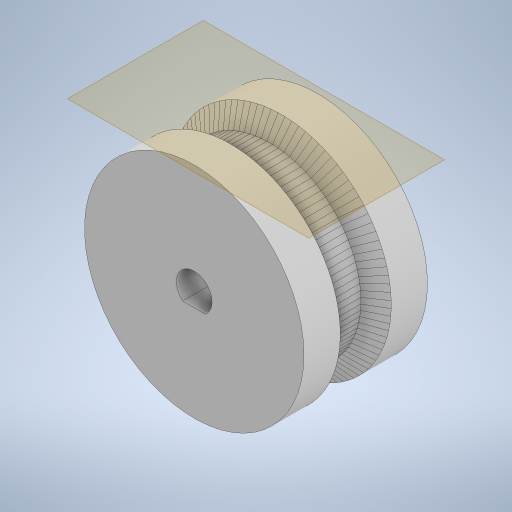
# Autodesk Inventor part: koło
Saved by Autodesk Inventor 2023 (Build 270158000, 158)
## iProperties
Created: 2022-12-13
Part Number: koło
Material: Generic
Document SubType Name: Modeling
Designer: komputer
Density: 1 g/cm^3
Appearance: Default
Author: komputer
Autodesk Inventor part; units mm, degrees
ref_plane "YZ Plane" through (0, 0, 0) normal (1, 0, 0) x (0, 1, 0)
ref_plane "XZ Plane" through (0, 0, 0) normal (0, 1, 0) x (-1, 0, 0)
ref_plane "XY Plane" through (0, 0, 0) normal (0, 0, 1) x (1, 0, 0)
sketch "Sketch1" plane through (0, 0, 0) normal (0, 0, 1) x (1, 0, 0)
  arc A0 (-0.4247, 0.01) -> (-2.6608, 0.01) centre (-1.5427, 1.01) ccw
  arc A1 (-2.6608, 0.01) -> (-0.4247, 0.01) centre (-1.5427, 1.01) ccw
  line L0 (-7.5427, -2.95) -> (-9.5427, -2.95)
  line L1 (-7.5427, 12.35) -> (-7.5427, -2.95)
  line L2 (-7.5427, 12.35) -> (-8.5427, 12.35)
  line L3 (-8.5427, 12.35) -> (-4.5427, 12.35)
  line L4 (-4.5427, 35.8608) -> (-4.5427, 12.35)
  line L5 (1.9573, 15.05) -> (-0.8499, 15.05)
  arc A2 (-2.2355, 15.05) -> (-0.8499, 15.05) centre (-1.5427, 13.95) ccw
  line L6 (-2.2355, 15.05) -> (-5.0427, 15.05)
  arc A3 (-5.0427, 15.05) -> (-5.5427, 14.55) centre (-5.0427, 14.55) ccw
  line L7 (-5.5427, 14.55) -> (-5.5427, 12.85)
  line L8 (-5.5427, 12.85) -> (-7.0427, 12.85)
  arc A4 (-7.0427, 12.85) -> (-7.5427, 12.35) centre (-7.0427, 12.35) ccw
  line L9 (-7.5427, 12.35) -> (-7.5427, -2.45)
  arc A5 (-7.5427, -2.45) -> (-7.0427, -2.95) centre (-7.0427, -2.45) ccw
  line L10 (-7.0427, -2.95) -> (3.9573, -2.95)
  arc A6 (3.9573, -2.95) -> (4.4573, -2.45) centre (3.9573, -2.45) ccw
  line L11 (4.4573, -2.45) -> (4.4573, 12.35)
  arc A7 (4.4573, 12.35) -> (3.9573, 12.85) centre (3.9573, 12.35) ccw
  line L12 (3.9573, 12.85) -> (2.4573, 12.85)
  line L13 (2.4573, 12.85) -> (2.4573, 14.55)
  arc A8 (2.4573, 14.55) -> (1.9573, 15.05) centre (1.9573, 14.55) ccw
  circle A9 centre (-1.5427, 1.01) radius 2
  circle A10 centre (1.2073, 9.85) radius 0.45
  circle A11 centre (0.0302, 6.6603) radius 0.45
  circle A12 centre (-1.5427, 4.59) radius 0.45
  circle A13 centre (2.7073, -1.24) radius 1.25
  circle A14 centre (-5.7927, -1.24) radius 1.25
  line L14 (-1.5427, 1.01) -> (-10.5427, 1.01)
  line L15 (-10.5427, 1.01) -> (-12.5427, 1.01)
  line L16 (-12.5427, 1.01) -> (-9.5427, 1.01)
  circle A15 centre (-1.5427, 1.01) radius 8
  line L17 (-1.5427, 1.01) -> (-1.5427, -6.99)
  line L18 (-1.5427, -6.99) -> (-1.5427, -9.99)
  line L19 (-2.3734, 0.01) -> (-0.7121, 0.01)
  arc A16 (-0.7121, 0.01) -> (-2.3734, 0.01) centre (-1.5427, 1.01) ccw
  line L20 (-8.5427, 12.35) -> (-8.5427, 10.01)
  line L21 (-8.5427, 10.01) -> (-11.5427, 10.01)
  line L22 (-8.5427, 36.4347) -> (-8.5427, 12.35)
  line L23 (-4.5427, 35.8608) -> (-8.5427, 36.4347)
  line L24 (-11.5427, 10.01) -> (-11.5427, -0.95)
  arc A17 (-11.5427, -0.95) -> (-9.5427, -2.95) centre (-9.5427, -0.95) ccw
  point P0 (0, 0)
extrude "Extrusion1" add sketch "Sketch1" against normal blind 9 contours A1 L17 L19 A16 L14 A0 | A0 L14 A9 L17 A1 | L14 A16 L19 L17 A1 A0 | A0 A1 L17 A9 L14 | L14 L1 A15 L11 A6 L10 L17 A9 | A9 L17 L10 A5 L1 L14 | L14 A15 L1 | L1 L0 A15 L14 | L17 A15 L0 L1 A5 L10 | L10 A6 L11 A15 L17 | A11 | A12 | A13 | A14
ref_plane "Płaszczyzna konstrukcyjna1" through (-1.5427, 9.01, 0) normal (0, 1, 0) x (1, 0, 0)
sketch "Szkic2" plane through (-1.5427, 9.01, 0) normal (0, 1, 0) x (1, 0, 0)
  line L0 (8, 9) -> (-8, 9) projected
  line L1 (-8, 0) -> (8, 0) projected
  line L2 (8, 0) -> (8, 9) projected
  line L3 (-8, 0) -> (-8, 9) projected
  line L4 (8, 4.5) -> (6.6434, 4.5)
  line L5 (6.6434, 4.5) -> (6.6434, 5.5)
  line L6 (6.6434, 5.5) -> (6.6434, 3.5)
  line L7 (6.6434, 3.5) -> (8, 2.6389)
  line L8 (6.6434, 5.5) -> (8, 6.3611)
  point P0 (1.5427, 0)
  dimension "d5" = 1
  dimension "d6" = 2
  constraints: 10 end point, 2 point on line, 1 horizontal, 1 midpoint, 1 perpendicular, 1 symmetric about line
  measures "d5" distance of L4.end L5.end
  measures "d6" distance of L5.end L6.end
extrude "Wyciągnięcie proste2" cut sketch "Szkic2" against normal through all contours L2 L4 L5 L8 | L2 L7 L6 L4
pattern_circular "Szyk kołowy1" count 100 over 360 about axis through (-1.5427, 1.01, 0) along (0, 0, -1) of "Wyciągnięcie proste2"
sketch "Szkic3" plane through (-2.3734, 0.01, 0) normal (0, 1, 0) x (1, 0, 0)
  line L0 (1.6613, 0) -> (0, 0) projected
  line L1 (1.6613, 0) -> (1.6613, 9) projected
  line L2 (0, 9) -> (1.6613, 9) projected
  line L3 (0, 0) -> (0, 9) projected
  ellipse E0 centre (0.8307, 1.283) end of major axis (8.8294, 6.356) minor radius 0.2693 (8.8267, 6.3586) -> (8.7952, 6.3586) ccw projected
  line L4 (8.8267, 6.3586) -> (8.8267, 6.3586) projected
  ellipse E1 centre (0.8307, 1.283) end of major axis (8.8294, 6.356) minor radius 0.2693 (8.8267, 6.3586) -> (8.7952, 6.3586) ccw projected
  ellipse E2 centre (0.8307, 1.283) end of major axis (8.8255, 6.3407) minor radius 0.5382 (8.7952, 6.3586) -> (8.7322, 6.3586) ccw projected
  ellipse E3 centre (0.8307, 1.283) end of major axis (8.8191, 6.3151) minor radius 0.8063 (8.7322, 6.3586) -> (8.638, 6.3586) ccw projected
  ellipse E4 centre (0.8307, 1.283) end of major axis (8.8104, 6.279) minor radius 1.0731 (8.638, 6.3586) -> (8.513, 6.3586) ccw projected
  ellipse E5 centre (0.8307, 1.283) end of major axis (8.7994, 6.2323) minor radius 1.3383 (8.513, 6.3586) -> (8.3577, 6.3586) ccw projected
  ellipse E6 centre (0.8307, 1.283) end of major axis (8.7866, 6.1745) minor radius 1.6013 (8.3577, 6.3586) -> (8.1727, 6.3586) ccw projected
  ellipse E7 centre (0.8307, 1.283) end of major axis (8.7721, 6.1054) minor radius 1.8617 (8.1727, 6.3586) -> (7.9587, 6.3586) ccw projected
  ellipse E8 centre (0.8307, 1.283) end of major axis (8.7563, 6.0244) minor radius 2.1191 (7.9587, 6.3586) -> (7.7166, 6.3586) ccw projected
  ellipse E9 centre (0.8307, 1.283) end of major axis (-7.0785, -3.3648) minor radius 2.3729 (7.7166, 6.3586) -> (7.4473, 6.3586) ccw projected
  ellipse E10 centre (0.8307, 1.283) end of major axis (-7.0617, -3.2579) minor radius 2.6225 (7.4473, 6.3586) -> (7.1519, 6.3586) ccw projected
  ellipse E11 centre (0.8307, 1.283) end of major axis (-7.0453, -3.1368) minor radius 2.8673 (7.1519, 6.3586) -> (6.8316, 6.3586) ccw projected
  ellipse E12 centre (0.8307, 1.283) end of major axis (-7.03, -3.0002) minor radius 3.1066 (6.8316, 6.3586) -> (6.4875, 6.3586) ccw projected
  ellipse E13 centre (0.8307, 1.283) end of major axis (-7.0167, -2.8465) minor radius 3.3396 (6.4875, 6.3586) -> (6.1212, 6.3586) ccw projected
  ellipse E14 centre (0.8307, 1.283) end of major axis (-7.0063, -2.6739) minor radius 3.5655 (6.1212, 6.3586) -> (5.7339, 6.3586) ccw projected
  ellipse E15 centre (0.8307, 1.283) end of major axis (-6.9997, -2.48) minor radius 3.7831 (5.7339, 6.3586) -> (5.3273, 6.3586) ccw projected
  ellipse E16 centre (0.8307, 1.283) end of major axis (-6.9981, -2.2621) minor radius 3.9912 (5.3273, 6.3586) -> (4.903, 6.3586) ccw projected
  ellipse E17 centre (0.8307, 1.283) end of major axis (-7.0023, -2.0168) minor radius 4.1884 (4.903, 6.3586) -> (4.4626, 6.3586) ccw projected
  ellipse E18 centre (0.8307, 1.283) end of major axis (-7.0133, -1.7401) minor radius 4.3727 (4.4626, 6.3586) -> (4.0078, 6.3586) ccw projected
  ellipse E19 centre (0.8307, 1.283) end of major axis (-7.0311, -1.4279) minor radius 4.5421 (4.0078, 6.3586) -> (3.5406, 6.3586) ccw projected
  ellipse E20 centre (0.8307, 1.283) end of major axis (-7.0554, -1.0759) minor radius 4.6938 (3.5406, 6.3586) -> (3.0626, 6.3586) ccw projected
  ellipse E21 centre (0.8307, 1.283) end of major axis (-7.0845, -0.6808) minor radius 4.825 (3.0626, 6.3586) -> (2.5758, 6.3586) ccw projected
  ellipse E22 centre (0.8307, 1.283) end of major axis (-7.1152, -0.2416) minor radius 4.9322 (2.5758, 6.3586) -> (2.0821, 6.3586) ccw projected
  ellipse E23 centre (0.8307, 1.283) end of major axis (-7.1428, 0.2388) minor radius 5.012 (2.0821, 6.3586) -> (1.5835, 6.3586) ccw projected
  ellipse E24 centre (0.8307, 1.283) end of major axis (-7.1623, 0.7518) minor radius 5.0614 (1.5835, 6.3586) -> (1.0819, 6.3586) ccw projected
  ellipse E25 centre (0.8307, 1.283) end of major axis (-7.1693, 1.283) minor radius 5.0781 (1.0819, 6.3586) -> (0.5794, 6.3586) ccw projected
  ellipse E26 centre (0.8307, 1.283) end of major axis (8.8236, 0.7518) minor radius 5.0614 (0.5794, 6.3586) -> (0.0778, 6.3586) ccw projected
  ellipse E27 centre (0.8307, 1.283) end of major axis (8.8041, 0.2388) minor radius 5.012 (0.0778, 6.3586) -> (-0.4208, 6.3586) ccw projected
  ellipse E28 centre (0.8307, 1.283) end of major axis (8.7765, -0.2416) minor radius 4.9322 (-0.4208, 6.3586) -> (-0.9145, 6.3586) ccw projected
  ellipse E29 centre (0.8307, 1.283) end of major axis (8.7458, -0.6808) minor radius 4.825 (-0.9145, 6.3586) -> (-1.4013, 6.3586) ccw projected
  ellipse E30 centre (0.8307, 1.283) end of major axis (8.7168, -1.0759) minor radius 4.6938 (-1.4013, 6.3586) -> (-1.8792, 6.3586) ccw projected
  ellipse E31 centre (0.8307, 1.283) end of major axis (8.6924, -1.4279) minor radius 4.5421 (-1.8792, 6.3586) -> (-2.3465, 6.3586) ccw projected
  ellipse E32 centre (0.8307, 1.283) end of major axis (8.6746, -1.7401) minor radius 4.3727 (-2.3465, 6.3586) -> (-2.8013, 6.3586) ccw projected
  ellipse E33 centre (0.8307, 1.283) end of major axis (8.6637, -2.0168) minor radius 4.1884 (-2.8013, 6.3586) -> (-3.2417, 6.3586) ccw projected
  ellipse E34 centre (0.8307, 1.283) end of major axis (8.6594, -2.2621) minor radius 3.9912 (-3.2417, 6.3586) -> (-3.666, 6.3586) ccw projected
  ellipse E35 centre (0.8307, 1.283) end of major axis (8.661, -2.48) minor radius 3.7831 (-3.666, 6.3586) -> (-4.0726, 6.3586) ccw projected
  ellipse E36 centre (0.8307, 1.283) end of major axis (8.6676, -2.6739) minor radius 3.5655 (-4.0726, 6.3586) -> (-4.4598, 6.3586) ccw projected
  ellipse E37 centre (0.8307, 1.283) end of major axis (8.678, -2.8465) minor radius 3.3396 (-4.4598, 6.3586) -> (-4.8262, 6.3586) ccw projected
  ellipse E38 centre (0.8307, 1.283) end of major axis (8.6914, -3.0002) minor radius 3.1066 (-4.8262, 6.3586) -> (-5.1702, 6.3586) ccw projected
  ellipse E39 centre (0.8307, 1.283) end of major axis (8.7066, -3.1368) minor radius 2.8673 (-5.1702, 6.3586) -> (-5.4906, 6.3586) ccw projected
  ellipse E40 centre (0.8307, 1.283) end of major axis (8.723, -3.2579) minor radius 2.6225 (-5.4906, 6.3586) -> (-5.786, 6.3586) ccw projected
  ellipse E41 centre (0.8307, 1.283) end of major axis (8.7398, -3.3648) minor radius 2.3729 (-5.786, 6.3586) -> (-6.0553, 6.3586) ccw projected
  ellipse E42 centre (0.8307, 1.283) end of major axis (8.7563, -3.4583) minor radius 2.1191 (-6.0553, 6.3586) -> (-6.2974, 6.3586) ccw projected
  ellipse E43 centre (0.8307, 1.283) end of major axis (8.7721, -3.5393) minor radius 1.8617 (-6.2974, 6.3586) -> (-6.5114, 6.3586) ccw projected
  ellipse E44 centre (0.8307, 1.283) end of major axis (8.7866, -3.6084) minor radius 1.6013 (-6.5114, 6.3586) -> (-6.6964, 6.3586) ccw projected
  ellipse E45 centre (0.8307, 1.283) end of major axis (8.7994, -3.6662) minor radius 1.3383 (-6.6964, 6.3586) -> (-6.8517, 6.3586) ccw projected
  ellipse E46 centre (0.8307, 1.283) end of major axis (8.8104, -3.713) minor radius 1.0731 (-6.8517, 6.3586) -> (-6.9767, 6.3586) ccw projected
  ellipse E47 centre (0.8307, 1.283) end of major axis (8.8191, -3.7491) minor radius 0.8063 (-6.9767, 6.3586) -> (-7.0708, 6.3586) ccw projected
  ellipse E48 centre (0.8307, 1.283) end of major axis (8.8255, -3.7747) minor radius 0.5382 (-7.0708, 6.3586) -> (-7.1338, 6.3586) ccw projected
  ellipse E49 centre (0.8307, 1.283) end of major axis (8.8294, -3.79) minor radius 0.2693 (-7.1338, 6.3586) -> (-7.1654, 6.3586) ccw projected
  line L5 (-7.1654, 6.3586) -> (-7.1654, 6.3586) projected
  ellipse E50 centre (0.8307, 1.283) end of major axis (8.8294, -3.79) minor radius 0.2693 (-7.1338, 6.3586) -> (-7.1654, 6.3586) ccw projected
  ellipse E51 centre (0.8307, 1.283) end of major axis (8.8255, -3.7747) minor radius 0.5382 (-7.0708, 6.3586) -> (-7.1338, 6.3586) ccw projected
  ellipse E52 centre (0.8307, 1.283) end of major axis (8.8191, -3.7491) minor radius 0.8063 (-6.9767, 6.3586) -> (-7.0708, 6.3586) ccw projected
  ellipse E53 centre (0.8307, 1.283) end of major axis (8.8104, -3.713) minor radius 1.0731 (-6.8517, 6.3586) -> (-6.9767, 6.3586) ccw projected
  ellipse E54 centre (0.8307, 1.283) end of major axis (8.7994, -3.6662) minor radius 1.3383 (-6.6964, 6.3586) -> (-6.8517, 6.3586) ccw projected
  ellipse E55 centre (0.8307, 1.283) end of major axis (8.7866, -3.6084) minor radius 1.6013 (-6.5114, 6.3586) -> (-6.6964, 6.3586) ccw projected
  ellipse E56 centre (0.8307, 1.283) end of major axis (8.7721, -3.5393) minor radius 1.8617 (-6.2974, 6.3586) -> (-6.5114, 6.3586) ccw projected
  ellipse E57 centre (0.8307, 1.283) end of major axis (8.7563, -3.4583) minor radius 2.1191 (-6.0553, 6.3586) -> (-6.2974, 6.3586) ccw projected
  ellipse E58 centre (0.8307, 1.283) end of major axis (-7.0785, 5.9308) minor radius 2.3729 (-5.786, 6.3586) -> (-6.0553, 6.3586) ccw projected
  ellipse E59 centre (0.8307, 1.283) end of major axis (-7.0617, 5.824) minor radius 2.6225 (-5.4906, 6.3586) -> (-5.786, 6.3586) ccw projected
  ellipse E60 centre (0.8307, 1.283) end of major axis (-7.0453, 5.7029) minor radius 2.8673 (-5.1702, 6.3586) -> (-5.4906, 6.3586) ccw projected
  ellipse E61 centre (0.8307, 1.283) end of major axis (-7.03, 5.5662) minor radius 3.1066 (-4.8262, 6.3586) -> (-5.1702, 6.3586) ccw projected
  ellipse E62 centre (0.8307, 1.283) end of major axis (-7.0167, 5.4125) minor radius 3.3396 (-4.4598, 6.3586) -> (-4.8262, 6.3586) ccw projected
  ellipse E63 centre (0.8307, 1.283) end of major axis (-7.0063, 5.2399) minor radius 3.5655 (-4.0726, 6.3586) -> (-4.4598, 6.3586) ccw projected
  ellipse E64 centre (0.8307, 1.283) end of major axis (-6.9997, 5.0461) minor radius 3.7831 (-3.666, 6.3586) -> (-4.0726, 6.3586) ccw projected
  ellipse E65 centre (0.8307, 1.283) end of major axis (-6.9981, 4.8282) minor radius 3.9912 (-3.2417, 6.3586) -> (-3.666, 6.3586) ccw projected
  ellipse E66 centre (0.8307, 1.283) end of major axis (-7.0023, 4.5828) minor radius 4.1884 (-2.8013, 6.3586) -> (-3.2417, 6.3586) ccw projected
  ellipse E67 centre (0.8307, 1.283) end of major axis (-7.0133, 4.3062) minor radius 4.3727 (-2.3465, 6.3586) -> (-2.8013, 6.3586) ccw projected
  ellipse E68 centre (0.8307, 1.283) end of major axis (-7.0311, 3.994) minor radius 4.5421 (-1.8792, 6.3586) -> (-2.3465, 6.3586) ccw projected
  ellipse E69 centre (0.8307, 1.283) end of major axis (-7.0554, 3.642) minor radius 4.6938 (-1.4013, 6.3586) -> (-1.8792, 6.3586) ccw projected
  ellipse E70 centre (0.8307, 1.283) end of major axis (-7.0845, 3.2469) minor radius 4.825 (-0.9145, 6.3586) -> (-1.4013, 6.3586) ccw projected
  ellipse E71 centre (0.8307, 1.283) end of major axis (-7.1152, 2.8076) minor radius 4.9322 (-0.4208, 6.3586) -> (-0.9145, 6.3586) ccw projected
  ellipse E72 centre (0.8307, 1.283) end of major axis (-7.1428, 2.3272) minor radius 5.012 (0.0778, 6.3586) -> (-0.4208, 6.3586) ccw projected
  ellipse E73 centre (0.8307, 1.283) end of major axis (-7.1623, 1.8142) minor radius 5.0614 (0.5794, 6.3586) -> (0.0778, 6.3586) ccw projected
  ellipse E74 centre (0.8307, 1.283) end of major axis (-7.1693, 1.283) minor radius 5.0781 (1.0819, 6.3586) -> (0.5794, 6.3586) ccw projected
  ellipse E75 centre (0.8307, 1.283) end of major axis (8.8236, 1.8142) minor radius 5.0614 (1.5835, 6.3586) -> (1.0819, 6.3586) ccw projected
  ellipse E76 centre (0.8307, 1.283) end of major axis (8.8041, 2.3272) minor radius 5.012 (2.0821, 6.3586) -> (1.5835, 6.3586) ccw projected
  ellipse E77 centre (0.8307, 1.283) end of major axis (8.7765, 2.8076) minor radius 4.9322 (2.5758, 6.3586) -> (2.0821, 6.3586) ccw projected
  ellipse E78 centre (0.8307, 1.283) end of major axis (8.7458, 3.2469) minor radius 4.825 (3.0626, 6.3586) -> (2.5758, 6.3586) ccw projected
  ellipse E79 centre (0.8307, 1.283) end of major axis (8.7168, 3.642) minor radius 4.6938 (3.5406, 6.3586) -> (3.0626, 6.3586) ccw projected
  ellipse E80 centre (0.8307, 1.283) end of major axis (8.6924, 3.994) minor radius 4.5421 (4.0078, 6.3586) -> (3.5406, 6.3586) ccw projected
  ellipse E81 centre (0.8307, 1.283) end of major axis (8.6746, 4.3062) minor radius 4.3727 (4.4626, 6.3586) -> (4.0078, 6.3586) ccw projected
  ellipse E82 centre (0.8307, 1.283) end of major axis (8.6637, 4.5828) minor radius 4.1884 (4.903, 6.3586) -> (4.4626, 6.3586) ccw projected
  ellipse E83 centre (0.8307, 1.283) end of major axis (8.6594, 4.8282) minor radius 3.9912 (5.3273, 6.3586) -> (4.903, 6.3586) ccw projected
  ellipse E84 centre (0.8307, 1.283) end of major axis (8.661, 5.0461) minor radius 3.7831 (5.7339, 6.3586) -> (5.3273, 6.3586) ccw projected
  ellipse E85 centre (0.8307, 1.283) end of major axis (8.6676, 5.2399) minor radius 3.5655 (6.1212, 6.3586) -> (5.7339, 6.3586) ccw projected
  ellipse E86 centre (0.8307, 1.283) end of major axis (8.678, 5.4125) minor radius 3.3396 (6.4875, 6.3586) -> (6.1212, 6.3586) ccw projected
  ellipse E87 centre (0.8307, 1.283) end of major axis (8.6914, 5.5662) minor radius 3.1066 (6.8316, 6.3586) -> (6.4875, 6.3586) ccw projected
  ellipse E88 centre (0.8307, 1.283) end of major axis (8.7066, 5.7029) minor radius 2.8673 (7.1519, 6.3586) -> (6.8316, 6.3586) ccw projected
  ellipse E89 centre (0.8307, 1.283) end of major axis (8.723, 5.824) minor radius 2.6225 (7.4473, 6.3586) -> (7.1519, 6.3586) ccw projected
  ellipse E90 centre (0.8307, 1.283) end of major axis (8.7398, 5.9308) minor radius 2.3729 (7.7166, 6.3586) -> (7.4473, 6.3586) ccw projected
  ellipse E91 centre (0.8307, 1.283) end of major axis (8.7563, 6.0244) minor radius 2.1191 (7.9587, 6.3586) -> (7.7166, 6.3586) ccw projected
  ellipse E92 centre (0.8307, 1.283) end of major axis (8.7721, 6.1054) minor radius 1.8617 (8.1727, 6.3586) -> (7.9587, 6.3586) ccw projected
  ellipse E93 centre (0.8307, 1.283) end of major axis (8.7866, 6.1745) minor radius 1.6013 (8.3577, 6.3586) -> (8.1727, 6.3586) ccw projected
  ellipse E94 centre (0.8307, 1.283) end of major axis (8.7994, 6.2323) minor radius 1.3383 (8.513, 6.3586) -> (8.3577, 6.3586) ccw projected
  ellipse E95 centre (0.8307, 1.283) end of major axis (8.8104, 6.279) minor radius 1.0731 (8.638, 6.3586) -> (8.513, 6.3586) ccw projected
  ellipse E96 centre (0.8307, 1.283) end of major axis (8.8191, 6.3151) minor radius 0.8063 (8.7322, 6.3586) -> (8.638, 6.3586) ccw projected
  ellipse E97 centre (0.8307, 1.283) end of major axis (8.8255, 6.3407) minor radius 0.5382 (8.7952, 6.3586) -> (8.7322, 6.3586) ccw projected
  line L6 (8.8307, 9) -> (-7.1693, 9) projected
  line L7 (-7.1693, 0) -> (8.8307, 0) projected
  ellipse E98 centre (0.8307, 7.717) end of major axis (8.8294, 2.644) minor radius 0.2693 (8.7952, 2.6414) -> (8.8267, 2.6414) ccw projected
  ellipse E99 centre (0.8307, 7.717) end of major axis (8.8255, 2.6593) minor radius 0.5382 (8.7322, 2.6414) -> (8.7952, 2.6414) ccw projected
  ellipse E100 centre (0.8307, 7.717) end of major axis (8.8191, 2.6849) minor radius 0.8063 (8.638, 2.6414) -> (8.7322, 2.6414) ccw projected
  ellipse E101 centre (0.8307, 7.717) end of major axis (8.8104, 2.721) minor radius 1.0731 (8.513, 2.6414) -> (8.638, 2.6414) ccw projected
  ellipse E102 centre (0.8307, 7.717) end of major axis (8.7994, 2.7677) minor radius 1.3383 (8.3577, 2.6414) -> (8.513, 2.6414) ccw projected
  ellipse E103 centre (0.8307, 7.717) end of major axis (8.7866, 2.8255) minor radius 1.6013 (8.1727, 2.6414) -> (8.3577, 2.6414) ccw projected
  ellipse E104 centre (0.8307, 7.717) end of major axis (8.7721, 2.8946) minor radius 1.8617 (7.9587, 2.6414) -> (8.1727, 2.6414) ccw projected
  ellipse E105 centre (0.8307, 7.717) end of major axis (8.7563, 2.9756) minor radius 2.1191 (7.7166, 2.6414) -> (7.9587, 2.6414) ccw projected
  ellipse E106 centre (0.8307, 7.717) end of major axis (-7.0785, 12.3648) minor radius 2.3729 (7.4473, 2.6414) -> (7.7166, 2.6414) ccw projected
  ellipse E107 centre (0.8307, 7.717) end of major axis (-7.0617, 12.2579) minor radius 2.6225 (7.1519, 2.6414) -> (7.4473, 2.6414) ccw projected
  ellipse E108 centre (0.8307, 7.717) end of major axis (-7.0453, 12.1368) minor radius 2.8673 (6.8316, 2.6414) -> (7.1519, 2.6414) ccw projected
  ellipse E109 centre (0.8307, 7.717) end of major axis (-7.03, 12.0002) minor radius 3.1066 (6.4875, 2.6414) -> (6.8316, 2.6414) ccw projected
  ellipse E110 centre (0.8307, 7.717) end of major axis (-7.0167, 11.8465) minor radius 3.3396 (6.1212, 2.6414) -> (6.4875, 2.6414) ccw projected
  ellipse E111 centre (0.8307, 7.717) end of major axis (-7.0063, 11.6739) minor radius 3.5655 (5.7339, 2.6414) -> (6.1212, 2.6414) ccw projected
  ellipse E112 centre (0.8307, 7.717) end of major axis (-6.9997, 11.48) minor radius 3.7831 (5.3273, 2.6414) -> (5.7339, 2.6414) ccw projected
  ellipse E113 centre (0.8307, 7.717) end of major axis (-6.9981, 11.2621) minor radius 3.9912 (4.903, 2.6414) -> (5.3273, 2.6414) ccw projected
  ellipse E114 centre (0.8307, 7.717) end of major axis (-7.0023, 11.0168) minor radius 4.1884 (4.4626, 2.6414) -> (4.903, 2.6414) ccw projected
  ellipse E115 centre (0.8307, 7.717) end of major axis (-7.0133, 10.7401) minor radius 4.3727 (4.0078, 2.6414) -> (4.4626, 2.6414) ccw projected
  ellipse E116 centre (0.8307, 7.717) end of major axis (-7.0311, 10.4279) minor radius 4.5421 (3.5406, 2.6414) -> (4.0078, 2.6414) ccw projected
  ellipse E117 centre (0.8307, 7.717) end of major axis (-7.0554, 10.0759) minor radius 4.6938 (3.0626, 2.6414) -> (3.5406, 2.6414) ccw projected
  ellipse E118 centre (0.8307, 7.717) end of major axis (-7.0845, 9.6808) minor radius 4.825 (2.5758, 2.6414) -> (3.0626, 2.6414) ccw projected
  ellipse E119 centre (0.8307, 7.717) end of major axis (-7.1152, 9.2416) minor radius 4.9322 (2.0821, 2.6414) -> (2.5758, 2.6414) ccw projected
  ellipse E120 centre (0.8307, 7.717) end of major axis (-7.1428, 8.7612) minor radius 5.012 (1.5835, 2.6414) -> (2.0821, 2.6414) ccw projected
  ellipse E121 centre (0.8307, 7.717) end of major axis (-7.1623, 8.2482) minor radius 5.0614 (1.0819, 2.6414) -> (1.5835, 2.6414) ccw projected
  ellipse E122 centre (0.8307, 7.717) end of major axis (8.8307, 7.717) minor radius 5.0781 (0.5794, 2.6414) -> (1.0819, 2.6414) ccw projected
  ellipse E123 centre (0.8307, 7.717) end of major axis (8.8236, 8.2482) minor radius 5.0614 (0.0778, 2.6414) -> (0.5794, 2.6414) ccw projected
  ellipse E124 centre (0.8307, 7.717) end of major axis (8.8041, 8.7612) minor radius 5.012 (-0.4208, 2.6414) -> (0.0778, 2.6414) ccw projected
  ellipse E125 centre (0.8307, 7.717) end of major axis (8.7765, 9.2416) minor radius 4.9322 (-0.9145, 2.6414) -> (-0.4208, 2.6414) ccw projected
  ellipse E126 centre (0.8307, 7.717) end of major axis (8.7458, 9.6808) minor radius 4.825 (-1.4013, 2.6414) -> (-0.9145, 2.6414) ccw projected
  ellipse E127 centre (0.8307, 7.717) end of major axis (8.7168, 10.0759) minor radius 4.6938 (-1.8792, 2.6414) -> (-1.4013, 2.6414) ccw projected
  ellipse E128 centre (0.8307, 7.717) end of major axis (8.6924, 10.4279) minor radius 4.5421 (-2.3465, 2.6414) -> (-1.8792, 2.6414) ccw projected
  ellipse E129 centre (0.8307, 7.717) end of major axis (8.6746, 10.7401) minor radius 4.3727 (-2.8013, 2.6414) -> (-2.3465, 2.6414) ccw projected
  ellipse E130 centre (0.8307, 7.717) end of major axis (8.6637, 11.0168) minor radius 4.1884 (-3.2417, 2.6414) -> (-2.8013, 2.6414) ccw projected
  ellipse E131 centre (0.8307, 7.717) end of major axis (8.6594, 11.2621) minor radius 3.9912 (-3.666, 2.6414) -> (-3.2417, 2.6414) ccw projected
  ellipse E132 centre (0.8307, 7.717) end of major axis (8.661, 11.48) minor radius 3.7831 (-4.0726, 2.6414) -> (-3.666, 2.6414) ccw projected
  ellipse E133 centre (0.8307, 7.717) end of major axis (8.6676, 11.6739) minor radius 3.5655 (-4.4598, 2.6414) -> (-4.0726, 2.6414) ccw projected
  ellipse E134 centre (0.8307, 7.717) end of major axis (8.678, 11.8465) minor radius 3.3396 (-4.8262, 2.6414) -> (-4.4598, 2.6414) ccw projected
  ellipse E135 centre (0.8307, 7.717) end of major axis (8.6914, 12.0002) minor radius 3.1066 (-5.1702, 2.6414) -> (-4.8262, 2.6414) ccw projected
  ellipse E136 centre (0.8307, 7.717) end of major axis (8.7066, 12.1368) minor radius 2.8673 (-5.4906, 2.6414) -> (-5.1702, 2.6414) ccw projected
  ellipse E137 centre (0.8307, 7.717) end of major axis (8.723, 12.2579) minor radius 2.6225 (-5.786, 2.6414) -> (-5.4906, 2.6414) ccw projected
  ellipse E138 centre (0.8307, 7.717) end of major axis (8.7398, 12.3648) minor radius 2.3729 (-6.0553, 2.6414) -> (-5.786, 2.6414) ccw projected
  ellipse E139 centre (0.8307, 7.717) end of major axis (8.7563, 12.4583) minor radius 2.1191 (-6.2974, 2.6414) -> (-6.0553, 2.6414) ccw projected
  ellipse E140 centre (0.8307, 7.717) end of major axis (8.7721, 12.5393) minor radius 1.8617 (-6.5114, 2.6414) -> (-6.2974, 2.6414) ccw projected
  ellipse E141 centre (0.8307, 7.717) end of major axis (8.7866, 12.6084) minor radius 1.6013 (-6.6964, 2.6414) -> (-6.5114, 2.6414) ccw projected
  ellipse E142 centre (0.8307, 7.717) end of major axis (8.7994, 12.6662) minor radius 1.3383 (-6.8517, 2.6414) -> (-6.6964, 2.6414) ccw projected
  ellipse E143 centre (0.8307, 7.717) end of major axis (8.8104, 12.713) minor radius 1.0731 (-6.9767, 2.6414) -> (-6.8517, 2.6414) ccw projected
  ellipse E144 centre (0.8307, 7.717) end of major axis (8.8191, 12.7491) minor radius 0.8063 (-7.0708, 2.6414) -> (-6.9767, 2.6414) ccw projected
  ellipse E145 centre (0.8307, 7.717) end of major axis (8.8255, 12.7747) minor radius 0.5382 (-7.1338, 2.6414) -> (-7.0708, 2.6414) ccw projected
  ellipse E146 centre (0.8307, 7.717) end of major axis (8.8294, 12.79) minor radius 0.2693 (-7.1654, 2.6414) -> (-7.1338, 2.6414) ccw projected
  line L8 (-7.1654, 2.6414) -> (-7.1654, 2.6414) projected
  ellipse E147 centre (0.8307, 7.717) end of major axis (8.8294, 12.79) minor radius 0.2693 (-7.1654, 2.6414) -> (-7.1338, 2.6414) ccw projected
  ellipse E148 centre (0.8307, 7.717) end of major axis (8.8255, 12.7747) minor radius 0.5382 (-7.1338, 2.6414) -> (-7.0708, 2.6414) ccw projected
  ellipse E149 centre (0.8307, 7.717) end of major axis (8.8191, 12.7491) minor radius 0.8063 (-7.0708, 2.6414) -> (-6.9767, 2.6414) ccw projected
  ellipse E150 centre (0.8307, 7.717) end of major axis (8.8104, 12.713) minor radius 1.0731 (-6.9767, 2.6414) -> (-6.8517, 2.6414) ccw projected
  ellipse E151 centre (0.8307, 7.717) end of major axis (8.7994, 12.6662) minor radius 1.3383 (-6.8517, 2.6414) -> (-6.6964, 2.6414) ccw projected
  ellipse E152 centre (0.8307, 7.717) end of major axis (8.7866, 12.6084) minor radius 1.6013 (-6.6964, 2.6414) -> (-6.5114, 2.6414) ccw projected
  ellipse E153 centre (0.8307, 7.717) end of major axis (8.7721, 12.5393) minor radius 1.8617 (-6.5114, 2.6414) -> (-6.2974, 2.6414) ccw projected
  ellipse E154 centre (0.8307, 7.717) end of major axis (8.7563, 12.4583) minor radius 2.1191 (-6.2974, 2.6414) -> (-6.0553, 2.6414) ccw projected
  ellipse E155 centre (0.8307, 7.717) end of major axis (-7.0785, 3.0692) minor radius 2.3729 (-6.0553, 2.6414) -> (-5.786, 2.6414) ccw projected
  ellipse E156 centre (0.8307, 7.717) end of major axis (-7.0617, 3.176) minor radius 2.6225 (-5.786, 2.6414) -> (-5.4906, 2.6414) ccw projected
  ellipse E157 centre (0.8307, 7.717) end of major axis (-7.0453, 3.2971) minor radius 2.8673 (-5.4906, 2.6414) -> (-5.1702, 2.6414) ccw projected
  ellipse E158 centre (0.8307, 7.717) end of major axis (-7.03, 3.4338) minor radius 3.1066 (-5.1702, 2.6414) -> (-4.8262, 2.6414) ccw projected
  ellipse E159 centre (0.8307, 7.717) end of major axis (-7.0167, 3.5875) minor radius 3.3396 (-4.8262, 2.6414) -> (-4.4598, 2.6414) ccw projected
  ellipse E160 centre (0.8307, 7.717) end of major axis (-7.0063, 3.7601) minor radius 3.5655 (-4.4598, 2.6414) -> (-4.0726, 2.6414) ccw projected
  ellipse E161 centre (0.8307, 7.717) end of major axis (-6.9997, 3.9539) minor radius 3.7831 (-4.0726, 2.6414) -> (-3.666, 2.6414) ccw projected
  ellipse E162 centre (0.8307, 7.717) end of major axis (-6.9981, 4.1718) minor radius 3.9912 (-3.666, 2.6414) -> (-3.2417, 2.6414) ccw projected
  ellipse E163 centre (0.8307, 7.717) end of major axis (-7.0023, 4.4172) minor radius 4.1884 (-3.2417, 2.6414) -> (-2.8013, 2.6414) ccw projected
  ellipse E164 centre (0.8307, 7.717) end of major axis (-7.0133, 4.6938) minor radius 4.3727 (-2.8013, 2.6414) -> (-2.3465, 2.6414) ccw projected
  ellipse E165 centre (0.8307, 7.717) end of major axis (-7.0311, 5.006) minor radius 4.5421 (-2.3465, 2.6414) -> (-1.8792, 2.6414) ccw projected
  ellipse E166 centre (0.8307, 7.717) end of major axis (-7.0554, 5.358) minor radius 4.6938 (-1.8792, 2.6414) -> (-1.4013, 2.6414) ccw projected
  ellipse E167 centre (0.8307, 7.717) end of major axis (-7.0845, 5.7531) minor radius 4.825 (-1.4013, 2.6414) -> (-0.9145, 2.6414) ccw projected
  ellipse E168 centre (0.8307, 7.717) end of major axis (-7.1152, 6.1924) minor radius 4.9322 (-0.9145, 2.6414) -> (-0.4208, 2.6414) ccw projected
  ellipse E169 centre (0.8307, 7.717) end of major axis (-7.1428, 6.6728) minor radius 5.012 (-0.4208, 2.6414) -> (0.0778, 2.6414) ccw projected
  ellipse E170 centre (0.8307, 7.717) end of major axis (-7.1623, 7.1858) minor radius 5.0614 (0.0778, 2.6414) -> (0.5794, 2.6414) ccw projected
  ellipse E171 centre (0.8307, 7.717) end of major axis (8.8307, 7.717) minor radius 5.0781 (0.5794, 2.6414) -> (1.0819, 2.6414) ccw projected
  ellipse E172 centre (0.8307, 7.717) end of major axis (8.8236, 7.1858) minor radius 5.0614 (1.0819, 2.6414) -> (1.5835, 2.6414) ccw projected
  ellipse E173 centre (0.8307, 7.717) end of major axis (8.8041, 6.6728) minor radius 5.012 (1.5835, 2.6414) -> (2.0821, 2.6414) ccw projected
  ellipse E174 centre (0.8307, 7.717) end of major axis (8.7765, 6.1924) minor radius 4.9322 (2.0821, 2.6414) -> (2.5758, 2.6414) ccw projected
  ellipse E175 centre (0.8307, 7.717) end of major axis (8.7458, 5.7531) minor radius 4.825 (2.5758, 2.6414) -> (3.0626, 2.6414) ccw projected
  ellipse E176 centre (0.8307, 7.717) end of major axis (8.7168, 5.358) minor radius 4.6938 (3.0626, 2.6414) -> (3.5406, 2.6414) ccw projected
  ellipse E177 centre (0.8307, 7.717) end of major axis (8.6924, 5.006) minor radius 4.5421 (3.5406, 2.6414) -> (4.0078, 2.6414) ccw projected
  ellipse E178 centre (0.8307, 7.717) end of major axis (8.6746, 4.6938) minor radius 4.3727 (4.0078, 2.6414) -> (4.4626, 2.6414) ccw projected
  ellipse E179 centre (0.8307, 7.717) end of major axis (8.6637, 4.4172) minor radius 4.1884 (4.4626, 2.6414) -> (4.903, 2.6414) ccw projected
  ellipse E180 centre (0.8307, 7.717) end of major axis (8.6594, 4.1718) minor radius 3.9912 (4.903, 2.6414) -> (5.3273, 2.6414) ccw projected
  ellipse E181 centre (0.8307, 7.717) end of major axis (8.661, 3.9539) minor radius 3.7831 (5.3273, 2.6414) -> (5.7339, 2.6414) ccw projected
  ellipse E182 centre (0.8307, 7.717) end of major axis (8.6676, 3.7601) minor radius 3.5655 (5.7339, 2.6414) -> (6.1212, 2.6414) ccw projected
  ellipse E183 centre (0.8307, 7.717) end of major axis (8.678, 3.5875) minor radius 3.3396 (6.1212, 2.6414) -> (6.4875, 2.6414) ccw projected
  ellipse E184 centre (0.8307, 7.717) end of major axis (8.6914, 3.4338) minor radius 3.1066 (6.4875, 2.6414) -> (6.8316, 2.6414) ccw projected
  ellipse E185 centre (0.8307, 7.717) end of major axis (8.7066, 3.2971) minor radius 2.8673 (6.8316, 2.6414) -> (7.1519, 2.6414) ccw projected
  ellipse E186 centre (0.8307, 7.717) end of major axis (8.723, 3.176) minor radius 2.6225 (7.1519, 2.6414) -> (7.4473, 2.6414) ccw projected
  ellipse E187 centre (0.8307, 7.717) end of major axis (8.7398, 3.0692) minor radius 2.3729 (7.4473, 2.6414) -> (7.7166, 2.6414) ccw projected
  ellipse E188 centre (0.8307, 7.717) end of major axis (8.7563, 2.9756) minor radius 2.1191 (7.7166, 2.6414) -> (7.9587, 2.6414) ccw projected
  ellipse E189 centre (0.8307, 7.717) end of major axis (8.7721, 2.8946) minor radius 1.8617 (7.9587, 2.6414) -> (8.1727, 2.6414) ccw projected
  ellipse E190 centre (0.8307, 7.717) end of major axis (8.7866, 2.8255) minor radius 1.6013 (8.1727, 2.6414) -> (8.3577, 2.6414) ccw projected
  ellipse E191 centre (0.8307, 7.717) end of major axis (8.7994, 2.7677) minor radius 1.3383 (8.3577, 2.6414) -> (8.513, 2.6414) ccw projected
  ellipse E192 centre (0.8307, 7.717) end of major axis (8.8104, 2.721) minor radius 1.0731 (8.513, 2.6414) -> (8.638, 2.6414) ccw projected
  ellipse E193 centre (0.8307, 7.717) end of major axis (8.8191, 2.6849) minor radius 0.8063 (8.638, 2.6414) -> (8.7322, 2.6414) ccw projected
  ellipse E194 centre (0.8307, 7.717) end of major axis (8.8255, 2.6593) minor radius 0.5382 (8.7322, 2.6414) -> (8.7952, 2.6414) ccw projected
  ellipse E195 centre (0.8307, 7.717) end of major axis (8.8294, 2.644) minor radius 0.2693 (8.7952, 2.6414) -> (8.8267, 2.6414) ccw projected
  line L9 (8.8267, 2.6414) -> (8.8267, 2.6414) projected
  line L10 (0, 6.36) -> (0, 2.64)
  line L11 (0, 4.5) -> (1.6613, 4.5)
  circle A0 centre (0.8307, 4.5) radius 1.25
  point P0 (2.3734, 0)
  dimension "d12" = 2.5
  constraints: 4 end point, 3 midpoint, 2 point on line, 1 centre point, 198 other
  measures "d12" diameter of A0
extrude "Wyciągnięcie proste3" cut sketch "Szkic3" along normal blind 1 and the other way blind 10 contours A0 L3 L11 L1 | L1 A0 | A0 L3 | L11 L3 A0 L1
sketch "Szkic4" plane through (-2.3734, 0.01, 0) normal (0, 1, 0) x (1, 0, 0)
  arc A0 (0, 3.5659) -> (1.6613, 3.5659) centre (0.8307, 4.5) ccw projected
  line L0 (0, 0) -> (0, 3.5659) projected
  line L1 (1.6613, 0) -> (0, 0) projected
  line L2 (1.6613, 0) -> (1.6613, 3.5659) projected
  circle A1 centre (0.8307, 4.5) radius 1.75
  point P0 (2.3734, 0)
  dimension "d17" = 3.5
  constraints: 1 centre point, 1 coincident
  measures "d17" diameter of A1
extrude "Wyciągnięcie proste4" cut sketch "Szkic4" along normal blind 2 and the other way blind 40 contours L0 A1 L2 A0 | A0 L2 A1 L0
body "Solid1"
